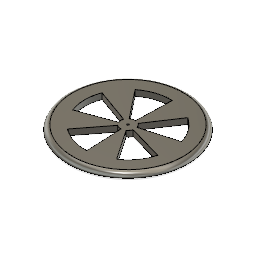
SkjotaraHjol1 v2 (Autodesk Fusion 360 design; units mm, degrees)
Autodesk Fusion 360 part; units mm, degrees
sketch "Sketch1" plane through (0, 0, 0) normal (0, 1, 0) x (1, 0, 0)
  circle A0 centre (0, 0) radius 100
  constraint coincident A0.centre origin
extrude "Extrude1" add sketch "Sketch1" along normal blind 10
form "Form1" [no effect]
sketch "Sketch2" plane through (0, 10, 0) normal (0, 1, 0) x (-1, 0, 0)
  circle A0 centre (0, 0) radius 1
  circle A1 centre (0, 0) radius 100
  dimension "d5" = 2
  constraint coincident A0.centre A1.centre
  measures "d5" diameter of A0
extrude "Extrude2" cut sketch "Sketch2" against normal blind 100 contours A0
sketch "Sketch3" plane through (0, 10, 0) normal (0, 1, 0) x (-1, 0, 0)
  circle A0 centre (0, 0) radius 1
  line L0 (-14.6615, 0) -> (28.0527, 0) construction
  line L1 (-14.6615, 0) -> (45.3385, 0) construction
  arc A1 (-69.209, -20.2512) -> (-40, -60) centre (0, 0) ccw
  line L2 (0, 0) -> (-69.209, -20.2512) construction
  line L3 (0, 0) -> (-40, -60) construction
  arc A2 (-11.6797, -3.4176) -> (-6.7504, -10.1256) centre (0, 0) ccw
  line L4 (-11.6797, -3.4176) -> (-69.209, -20.2512)
  line L5 (-6.7504, -10.1256) -> (-40, -60)
  circle A3 centre (0, 0) radius 100
  dimension "d12" = 40
  constraint horizontal L0
  constraint horizontal L1
  constraint coincident A0.centre A1.centre
  constraint coincident L2 A2.start
  constraint coincident L3 A2.end
  measures "d12" angle of L2 L3
extrude "Extrude3" cut sketch "Sketch3" against normal blind 70 contours A1 A2 L4 L5
pattern_circular "C-Pattern1" count 5 over 360 about axis through (0, 10, 0) along (0, -1, 0) of "Extrude3"
move_face "OffsetFaces1" offset -0.55 1 faces at (-0.995, 6.6667, -0.0996)
fillet "Fillet3" radius 7.5 1 edges at (-93.2327, 10, 36.1615)
fillet "Fillet4" radius 7.5 1 edges at (-93.2327, 0, 36.1615)
